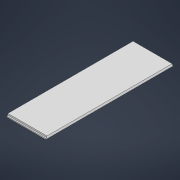
# Autodesk Inventor part: top
Saved by Autodesk Inventor 2022 (Build 260153000, 153)
## iProperties
Created: 2022-10-10
Part Number: top
Material: 常规
Document SubType Name: Modeling
Designer: 15628
Density: 1 g/cm^3
Appearance: 默认
Author: 15628
Autodesk Inventor part; units mm, degrees
ref_plane "YZ Plane" through (0, 0, 0) normal (1, 0, 0) x (0, 1, 0)
ref_plane "XZ Plane" through (0, 0, 0) normal (0, 1, 0) x (-1, 0, 0)
ref_plane "XY Plane" through (0, 0, 0) normal (0, 0, 1) x (1, 0, 0)
sketch "草图1" plane through (0, 0, 0) normal (0, 1, 0) x (-1, 0, 0)
  line L0 (0, 0) -> (28.2, 0)
  line L1 (28.2, 0) -> (28.2, -92.2)
  line L2 (28.2, -92.2) -> (0, -92.2)
  line L3 (0, -92.2) -> (0, 0)
  dimension "d0" = 28.2
  dimension "d1" = 92.2
  constraints: 8 end point, 2 parallel, 1 horizontal, 1 perpendicular
  measures "d0" distance of L1.end L2.end
  measures "d1" distance of L0.end L1.end
extrude "拉伸1" add sketch "草图1" along normal blind 1.8
sketch "草图2" plane through (0, 0, 0) normal (1, 0, 0) x (0, 0, -1)
  line L0 (0, 0) -> (0, 1.8) projected
  line L1 (0, 1.8) -> (0.9, 1.8)
  line L2 (0.9, 1.8) -> (0.9, 0.9)
  line L3 (0.9, 0.9) -> (0, 0.9)
  line L4 (0, 0.9) -> (0, 1.8)
  line L5 (92.2, 0) -> (0, 0) projected
  line L6 (0, 0) -> (0.9, 0)
  line L7 (0.9, 0) -> (0.9, 0.64)
  line L8 (0.9, 0.64) -> (0, 0.64)
  line L9 (0, 0.64) -> (0, 0)
  line L10 (92.2, 1.8) -> (0, 1.8) projected
  line L11 (0, 1.8) -> (0.9, 1.8)
  line L12 (0.9, 1.8) -> (0.9, 0.64)
  line L13 (0.9, 0.64) -> (0, 0.64)
  line L14 (0, 0.64) -> (0, 1.8)
  line L15 (92.2, 1.8) -> (91.3, 1.8)
  line L16 (91.3, 1.8) -> (91.3, 0.64)
  line L17 (91.3, 0.64) -> (92.2, 0.64)
  line L18 (92.2, 0.64) -> (92.2, 1.8)
  line L19 (91.3, 0.64) -> (92.2, 0.64)
  line L20 (92.2, 0.64) -> (92.2, 0)
  line L21 (92.2, 0) -> (91.3, 0)
  line L22 (91.3, 0) -> (91.3, 0.64)
  dimension "d4" = 0.9
  dimension "d5" = 0.64
  dimension "d6" = 0.9
  constraints: 40 end point, 10 parallel, 5 horizontal, 5 perpendicular, 1 point on line
  measures "d4" distance of L2.end L3.end
  measures "d5" distance of L7.end L6.end
  measures "d6" distance of L17.end L16.end
extrude "拉伸2" cut sketch "草图2" against normal through all contours L0 L3 L12 L8 | L0 L1 L2 L3 | L16 L10 L18 L17
